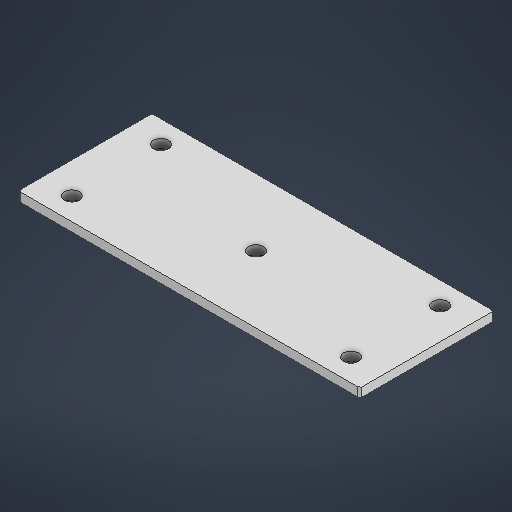
# Autodesk Inventor part: rig_connector
Saved by Autodesk Inventor 2027.1 (Build 311270010, 270A)
## iProperties
Created: 2026-09-04
Part Number: rig_connector
Material: Generic
Document SubType Name: Modeling
Designer: ajrcr
Density: 1 g/cm^3
Appearance: Default
Author: ajrcr
Autodesk Inventor part; units mm, degrees
ref_plane "YZ Plane" through (0, 0, 0) normal (1, 0, 0) x (0, 1, 0)
ref_plane "XZ Plane" through (0, 0, 0) normal (0, 1, 0) x (-1, 0, 0)
ref_plane "XY Plane" through (0, 0, 0) normal (0, 0, 1) x (1, 0, 0)
sketch "Sketch1" plane through (0, 0, 0) normal (0, 1, 0) x (-1, 0, 0)
  line L0 (-113.5, -45) -> (113.5, -45)
  line L1 (115, -44) -> (115, 44)
  line L2 (113.5, 45) -> (-113.5, 45)
  line L3 (-115, 44) -> (-115, -44)
  circle A0 centre (0, 0) radius 5
  line L4 (-113.5, -45) -> (-115, -44)
  line L5 (-115, 44) -> (-113.5, 45)
  line L6 (115, 44) -> (113.5, 45)
  line L7 (115, -44) -> (113.5, -45)
  circle A1 centre (-94, -30) radius 5
  circle A2 centre (-94, 30) radius 5
  line L8 (0, 45) -> (0, -45) construction
  circle A3 centre (94, -30) radius 5
  circle A4 centre (94, 30) radius 5
  point P0 (-115, -45)
  point P1 (115, 45)
  point P2 (115, -45)
  point P3 (-115, 45)
  point P4 (115, 0)
  dimension "d0" = 230
  dimension "d1" = 90
  dimension "d2" = 115
  dimension "d3" = 45
  dimension "d6" = 10
  dimension "d7" = 1.5
  dimension "d8" = 1
  dimension "d9" = 1
  dimension "d10" = 1.5
  dimension "d11" = 1
  dimension "d12" = 1.5
  dimension "d13" = 1
  dimension "d14" = 1.5
  dimension "d15" = 10
  dimension "d16" = 10
  dimension "d17" = 30
  dimension "d18" = 30
  dimension "d19" = 94
  dimension "d20" = 94
  constraints: 18 end point, 8 point on line, 5 centre point, 3 midpoint, 2 parallel, 2 symmetric about line, 1 coincident, 1 horizontal, 1 perpendicular, 2 other
  measures "d0" distance of point (-115, 45) point (115, 45)
  measures "d1" distance of point (115, 45) point (115, -45)
  measures "d2" distance of point (0, 0) point (115, 0)
  measures "d3" distance from line of L0 point (0, 0)
  measures "d6" diameter of A0
  measures "d7" distance of L0.start point (-115, -45)
  measures "d8" distance of L3.end point (-115, -45)
  measures "d9" distance of L3.start point (-115, 45)
  measures "d10" distance of L2.end point (-115, 45)
  measures "d11" distance of L1.end point (115, 45)
  measures "d12" distance of L2.start point (115, 45)
  measures "d13" distance of L1.start point (115, -45)
  measures "d14" distance of L0.end point (115, -45)
  measures "d15" diameter of A1
  measures "d16" diameter of A2
  measures "d17" vertical distance of point (0, 0) A1.centre
  measures "d18" vertical distance of point (0, 0) A2.centre
  measures "d19" horizontal distance of point (0, 0) A1.centre
  measures "d20" horizontal distance of point (0, 0) A2.centre
extrude "Extrusion1" add sketch "Sketch1" along normal blind 6
equation "\"d2\" = 0.5 * d0"
equation "\"d3\" = 0.5 * d1"
equation "\"d9\" = d8"
equation "\"d10\" = d7"
equation "\"d11\" = d8"
equation "\"d12\" = d7"
equation "\"d13\" = d8"
equation "\"d14\" = d7"
equation "\"d18\" = d17"
equation "\"d19\" = plate_thick + 0.5 * plates_spacing + brakcet_hole_to_plate"
equation "\"d20\" = d19"
equation "\"plate_thick\" = 6"
equation "\"plates_spacing\" = 116"
equation "\"brakcet_hole_to_plate\" = 30"
body "Solid1"
